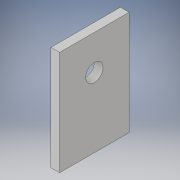
# Autodesk Inventor part: StressTestPlate
Saved by Autodesk Inventor 2017 (Build 210142000, 142)
## iProperties
Created: 2018-03-21
Part Number: StressTestPlate
Material: Generic
Document SubType Name: Modeling
Designer: User
Density: 1 g/cm^3
Appearance: Default
Mass: 23.7762 g
Surface Area: 93.5482 cm^2
Volume: 23.7762 cm^3
Author: User
Autodesk Inventor part; units mm, degrees
ref_plane "YZ Plane" through (0, 0, 0) normal (1, 0, 0) x (0, 1, 0)
ref_plane "XZ Plane" through (0, 0, 0) normal (0, 1, 0) x (-1, 0, 0)
ref_plane "XY Plane" through (0, 0, 0) normal (0, 0, 1) x (1, 0, 0)
sketch "Sketch1" plane through (0, 0, 0) normal (1, 0, 0) x (0, 1, 0)
  line L0 (0, 0) -> (-76.2, 0)
  line L1 (-76.2, 0) -> (-76.2, -50.8)
  line L2 (-76.2, -50.8) -> (0, -50.8)
  line L3 (0, -50.8) -> (0, 0)
  dimension "d0" = 76.2
  dimension "d1" = 50.8
  constraints: 8 end point, 2 parallel, 1 horizontal, 1 perpendicular
  measures "d0" distance of L2.end L1.end
  measures "d1" distance of L1.end L0.end
extrude "Extrusion1" add sketch "Sketch1" along normal blind 6.35
sketch "Sketch2" plane through (0, 0, 0) normal (-1, 0, 0) x (0, 0, 1)
  line L0 (-50.8, -76.2) -> (-50.8, 0) projected
  line L1 (0, 0) -> (0, -76.2) projected
  line L2 (-50.8, 0) -> (0, 0) projected
  point P0 (-25.4, -25.4)
  dimension "d4" = 50.8
  dimension "d5" = 25.4
  dimension "d6" = 25.4
  measures "d4" distance between parallel lines of L0 L1
  measures "d5" distance from line of L1 point (-25.4, -25.4)
  measures "d6" distance from line of L2 point (-25.4, -25.4)
hole "Hole1" at (0, -25.4, -25.4) direction (1, 0, 0) diameter 12.7 depth 25.4 tip angle 118
equation "\"d5\" = 0.5 * d4"
equation "\"d6\" = d5"
body "Solid1"
